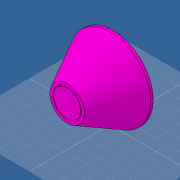
# Autodesk Inventor part: Zyklon_Konus
Saved by Autodesk Inventor 2019 (Build 230136000, 136)
## iProperties
Created: 2020-08-01
Part Number: Zyklon_Konus
Material: Generisch
Document SubType Name: Modeling
Designer: Stefan
Mass: 675.278 g
Surface Area: 698.059 cm^2
Volume: 675.278 cm^3
Density: 1 g/cm^3
Appearance: Magenta
Author: Stefan
Autodesk Inventor part; units mm, degrees
ref_plane "YZ Plane" through (0, 0, 0) normal (1, 0, 0) x (0, 1, 0)
ref_plane "XZ Plane" through (0, 0, 0) normal (0, 1, 0) x (-1, 0, 0)
ref_plane "XY Plane" through (0, 0, 0) normal (0, 0, 1) x (1, 0, 0)
sketch "Skizze1" plane through (0, 0, 0) normal (0, 0, 1) x (1, 0, 0)
  circle A0 centre (0, 0) radius 70
  circle A1 centre (0, 0) radius 25.05
  circle A2 centre (0, 0) radius 23.05
  dimension "d0" = 140
  dimension "d1" = 50.1
  dimension "d2" = 46.1
  constraints: 3 centre point, 3 coincident
  measures "d0" diameter of A0
  measures "d1" diameter of A1
  measures "d2" diameter of A2
extrude "Extrusion1" add sketch "Skizze1" against normal blind 5 contours A0 | A1 | A2
extrude "Extrusion2" add sketch "Skizze1" along normal blind 75
sketch "Skizze2" plane through (0, 0, 0) normal (1, 0, 0) x (0, 1, 0)
  line L0 (23.05, 75) -> (23.05, 0) projected
  line L1 (23.05, 0) -> (25.05, 0) projected
  line L2 (25.05, 0) -> (25.05, 75) projected
  line L3 (25.05, 75) -> (70, 75) projected
  line L4 (70, 75) -> (70, -5) projected
  line L5 (70, -5) -> (-70, -5) projected
  line L6 (-70, -5) -> (-70, 75) projected
  line L7 (-70, 75) -> (-25.05, 75) projected
  line L8 (-25.05, 75) -> (-25.05, 0) projected
  line L9 (-25.05, 0) -> (-23.05, 0) projected
  line L10 (-23.05, 0) -> (-23.05, 75) projected
  line L11 (-23.05, 75) -> (23.05, 75) projected
  line L12 (70, 75) -> (70, 0)
  line L13 (0, 75) -> (0, -5) construction
  line L14 (70, 0) -> (30.05, 75)
  line L15 (70, 75) -> (30.05, 75)
  point P0 (0, 0)
  dimension "d7" = 5
  constraints: 8 end point, 2 collinear, 2 midpoint, 2 point on line, 1 horizontal alignment
  measures "d7" distance from line of L14.end L2
revolve "Umdrehung1" cut sketch "Skizze2" angle 360 about axis through (0, 0, 75) along (0, 0, -1) contours L3 L4 L14
